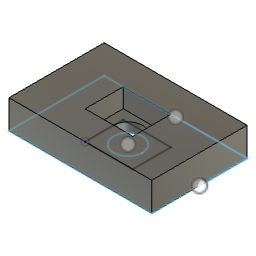
screw_holder_for_boat (Autodesk Fusion 360 design; units mm, degrees)
Autodesk Fusion 360 part; units mm, degrees
sketch "Sketch1" plane through (0, 0, 0) normal (0, 0, 1) x (1, 0, 0)
  line L0 (0, 0) -> (10, 0)
  line L1 (10, 0) -> (10, 8)
  line L2 (10, 8) -> (0, 8)
  line L3 (0, 8) -> (0, 0)
  circle A0 centre (5, 4) radius 3
  line L4 (20, 4) -> (20, 14)
  line L5 (20, 14) -> (5, 14)
  line L6 (20, 14) -> (-10, 14)
  line L7 (-10, 14) -> (-10, -6)
  line L8 (-10, -6) -> (20, -6)
  line L9 (20, -6) -> (20, 14)
  dimension "d3" = 10
  dimension "d4" = 8
  dimension "d5" = 6
  dimension "d6" = 15
  dimension "d7" = 10
  dimension "d8" = 30
  dimension "d9" = 20
  constraint horizontal L0
  constraint vertical L1
  constraint horizontal L2
  constraint vertical L3
  constraint coincident L0.start L3.end
  constraint vertical L4
  constraint horizontal L5
  constraint horizontal L6
  constraint vertical L7
  constraint horizontal L8
  constraint vertical L9
  measures "d3" distance of L0.start L0.end
  measures "d4" distance of L0.start L2.end
  measures "d5" diameter of A0
  measures "d6" distance of A0.centre L4.start
  measures "d7" distance of A0.centre L5.end
  measures "d8" distance of L4.end L6.end
  measures "d9" distance of L4.end L8.end
extrude "Extrude1" add sketch "Sketch1" along normal blind 6 contours L4 L5 L6 L7 L8 L9
extrude "Extrude2" add sketch "Sketch1" along normal blind 2 contours L0 L1 L2 L3
